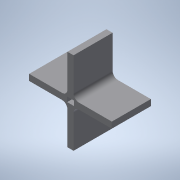
# Autodesk Inventor part: windmillv3
Saved by Autodesk Inventor 2022 (Build 260153000, 153)
## iProperties
Created: 2021-11-28
Part Number: windmillv3
Material: Generic
Document SubType Name: Modeling
Designer: haibo
Density: 1 g/cm^3
Appearance: Default
Author: haibo
Autodesk Inventor part; units mm, degrees
ref_plane "YZ Plane" through (0, 0, 0) normal (1, 0, 0) x (0, 1, 0)
ref_plane "XZ Plane" through (0, 0, 0) normal (0, 1, 0) x (-1, 0, 0)
ref_plane "XY Plane" through (0, 0, 0) normal (0, 0, 1) x (1, 0, 0)
sketch "Sketch1" plane through (0, 0, 0) normal (0, 0, 1) x (1, 0, 0)
  circle A0 centre (0, 0) radius 7.499998
  dimension "d0" = 15
  constraints: 1 centre point, 1 coincident
  measures "d0" diameter of A0
extrude "Extrusion1" add sketch "Sketch1" along normal blind 9.99998 and the other way blind 28.10002
sketch "Sketch2" plane through (0, 0, 9.99998) normal (0, 0, 1) x (1, 0, 0)
  line L0 (-2.778125, -1.984375) -> (2.778125, -1.984375)
  line L1 (2.778125, -1.984375) -> (2.778125, 1.984375)
  line L2 (2.778125, 1.984375) -> (-2.778125, 1.984375)
  line L3 (-2.778125, 1.984375) -> (-2.778125, -1.984375)
  line L4 (-2.778125, -1.984375) -> (2.778125, 1.984375) construction
  line L5 (2.778125, -1.984375) -> (-2.778125, 1.984375) construction
  point P0 (0, 0)
  dimension "d3" = 5.55625
  dimension "d4" = 3.96875
  constraints: 12 end point, 2 midpoint, 2 parallel, 1 horizontal, 1 perpendicular
  measures "d3" distance of L2.end L1.end
  measures "d4" distance of L1.end L0.end
extrude "Extrusion2" cut sketch "Sketch2" against normal blind 7.9375
ref_plane "Work Plane1" through (0, 0, 0) normal (0, 1, 0) x (0, 0, 1)
ref_plane "Work Plane2" through (0, 0, 0) normal (-1, 0, 0) x (0, 0, 1)
sketch "Sketch3" plane through (0, 0, 0) normal (0, 1, 0) x (0, 0, 1)
  point P0 (0, 0)
ref_plane "Work Plane3" through (0, 7.499998, 0) normal (0, 1, 0) x (-1, 0, 0)
ref_plane "Work Plane4" through (0, -7.499998, 0) normal (0, 1, 0) x (-1, 0, 0)
ref_plane "Work Plane5" through (-7.499998, 0, 0) normal (-1, 0, 0) x (0, -1, 0)
ref_plane "Work Plane6" through (7.499998, 0, 0) normal (-1, 0, 0) x (0, -1, 0)
sketch "Sketch4" plane through (0, 7.499998, 0) normal (0, 1, 0) x (-1, 0, 0)
  point P0 (0, 0)
sketch "Sketch5" plane through (0, 7.499998, 0) normal (0, 1, 0) x (-1, 0, 0)
  line L0 (7.499998, 9.99998) -> (-7.499998, 9.99998)
  line L1 (-2.534779, 9.99998) -> (2.534779, 9.99998)
  line L2 (2.534779, 9.99998) -> (2.534779, -28.099834)
  line L3 (2.534779, -28.099834) -> (-2.534779, -28.099834)
  line L4 (-2.534779, -28.099834) -> (-2.534779, 9.99998)
  point P0 (0, 0)
  constraints: 8 end point, 2 parallel, 2 point on line, 1 perpendicular
sketch "Sketch6" plane through (7.499998, 0, 0) normal (-1, 0, 0) x (0, -1, 0)
  line L0 (-2.534779, 9.99998) -> (2.534779, 9.99998)
  line L1 (2.534779, 9.99998) -> (2.534779, -28.099834)
  line L2 (2.534779, -28.099834) -> (-2.534779, -28.099834)
  line L3 (-2.534779, -28.099834) -> (-2.534779, 9.99998)
  point P0 (0, 0)
  constraints: 8 end point, 2 parallel, 1 perpendicular
sketch "Sketch7" plane through (0, -7.499998, 0) normal (0, 1, 0) x (-1, 0, 0)
  point P0 (0, 0)
sketch "Sketch8" plane through (0, -7.499998, 0) normal (0, 1, 0) x (-1, 0, 0)
  line L0 (-2.534779, 9.99998) -> (2.534779, 9.99998)
  line L1 (2.534779, 9.99998) -> (2.534779, -28.099834)
  line L2 (2.534779, -28.099834) -> (-2.534779, -28.099834)
  line L3 (-2.534779, -28.099834) -> (-2.534779, 9.99998)
  point P0 (0, 0)
  constraints: 8 end point, 2 parallel, 1 perpendicular
sketch "Sketch9" plane through (0, -7.499998, 0) normal (0, 1, 0) x (-1, 0, 0)
  point P0 (0, 0)
sketch "Sketch10" plane through (-7.499998, 0, 0) normal (-1, 0, 0) x (0, -1, 0)
  line L0 (7.499998, 9.99998) -> (-7.499998, 9.99998)
  line L1 (-2.542169, 9.99998) -> (2.537831, 9.99998)
  line L2 (2.537831, 9.99998) -> (2.537831, -28.10002)
  line L3 (2.537831, -28.10002) -> (-2.542169, -28.10002)
  line L4 (-2.542169, -28.10002) -> (-2.542169, 9.99998)
  point P0 (0, 0)
  dimension "d9" = 5.08
  dimension "d10" = 38.1
  constraints: 8 end point, 2 parallel, 2 point on line, 1 perpendicular
  measures "d9" distance of L1.start L1.end
  measures "d10" distance of L1.end L2.end
extrude "Extrusion3" add sketch "Sketch5" along normal blind 26.67 and the other way blind 1.27
extrude "Extrusion4" add sketch "Sketch6" along normal blind 1.27 and the other way blind 26.67
extrude "Extrusion5" add sketch "Sketch10" along normal blind 26.67 and the other way blind 1.27
extrude "Extrusion6" add sketch "Sketch8" along normal blind 1.27 and the other way blind 26.67
sketch "Sketch11" plane through (0, 0, 9.99998) normal (0, 0, 1) x (1, 0, 0)
  line L0 (2.534779, 7.058673) -> (2.534779, 6.979779)
  line L1 (34.169998, 2.534779) -> (7.058673, 2.534779)
  line L2 (6.979779, 2.534779) -> (7.058673, 2.534779)
  arc A0 (2.534779, 6.979779) -> (6.979779, 2.534779) centre (6.979779, 6.979779) ccw
  arc A1 (7.058673, 2.534779) -> (2.534779, 7.058673) centre (0, 0) ccw
  arc A2 (7.058673, 2.534779) -> (2.534779, 7.058673) centre (0, 0) ccw
  arc A3 (-2.534779, 7.058673) -> (-7.058673, 2.534779) centre (0, 0) ccw
  arc A4 (-6.979779, 2.534779) -> (-2.534779, 6.979779) centre (-6.979779, 6.979779) ccw
  line L3 (-7.058673, 2.534779) -> (-6.979779, 2.534779)
  line L4 (-2.534779, 6.979779) -> (-2.534779, 7.058673)
  arc A5 (-7.058673, -2.534779) -> (-2.534779, -7.058673) centre (0, 0) ccw
  arc A6 (-2.534779, -6.979779) -> (-6.979779, -2.534779) centre (-6.979779, -6.979779) ccw
  line L5 (-2.534779, -7.058673) -> (-2.534779, -6.979779)
  line L6 (-6.979779, -2.534779) -> (-7.058673, -2.534779)
  arc A7 (2.534779, -7.058673) -> (7.058673, -2.534779) centre (0, 0) ccw
  arc A8 (6.979779, -2.534779) -> (2.534779, -6.979779) centre (6.979779, -6.979779) ccw
  line L7 (7.058673, -2.534779) -> (6.979779, -2.534779)
  line L8 (2.534779, -6.979779) -> (2.534779, -7.058673)
  dimension "d29" = 4.445
  dimension "d32" = 360
  constraints: 16 end point, 16 point on circle, 8 centre point, 2 perpendicular, 2 tangent, 1 concentric, 41 other
  measures "d29" radius of A0
extrude "Extrusion7" cut sketch "Sketch11" against normal blind 38.1
sketch "Sketch12" plane through (0, 0, -28.10002) normal (0, 0, -1) x (-1, 0, 0)
  line L0 (2.534779, 7.058673) -> (2.534779, 34.169998)
  line L1 (-2.534779, 34.169998) -> (2.534779, 34.169998)
  line L2 (-2.534779, 7.058673) -> (-2.534779, 34.169998)
  arc A0 (-6.979779, 2.534779) -> (-2.534779, 6.979779) centre (-6.979779, 6.979779) ccw
  line L3 (-34.169998, 2.534779) -> (-7.058673, 2.534779)
  line L4 (-34.169998, -2.534779) -> (-34.169998, 2.534779)
  line L5 (-34.169998, -2.534779) -> (-7.058673, -2.534779)
  arc A1 (-2.534779, -6.979779) -> (-6.979779, -2.534779) centre (-6.979779, -6.979779) ccw
  line L6 (-2.534779, -34.169998) -> (-2.534779, -7.058673)
  line L7 (2.534779, -34.169998) -> (-2.534779, -34.169998)
  line L8 (2.534779, -34.169998) -> (2.534779, -7.058673)
  arc A2 (6.979779, -2.534779) -> (2.534779, -6.979779) centre (6.979779, -6.979779) ccw
  line L9 (7.057576, -2.537831) -> (34.169998, -2.537831)
  line L10 (34.169998, 2.542169) -> (34.169998, -2.537831)
  line L11 (7.056015, 2.542169) -> (34.169998, 2.542169)
  arc A3 (2.534779, 6.979779) -> (6.979779, 2.534779) centre (6.979779, 6.979779) ccw
  point P0 (0, 0)
extrude "Extrusion8" cut sketch "Sketch12" against normal blind 5.842 fills toward (2.484779, 20.614335) open curves L0 L1 L2
sketch "Sketch13" plane through (34.169998, 2.534779, -28.099834) normal (0, 0, -1) x (-1, 0, 0)
  line L0 (0, 0) -> (27.111325, 0)
  arc A0 (27.111325, 0) -> (27.111325, -5.069558) centre (34.169998, -2.534779) ccw
  line L1 (0, 0) -> (27.111325, 0)
  line L2 (0, -5.069558) -> (0, 0)
  line L3 (0, -5.069558) -> (27.111325, -5.069558)
  line L4 (31.635219, -9.514558) -> (31.635219, 4.445)
  arc A1 (27.190219, 0) -> (31.635219, 4.445) centre (27.190219, 4.445) ccw
  line L5 (27.190219, 0) -> (27.111325, 0)
  arc A2 (27.111325, 0) -> (27.111325, -5.069558) centre (34.169998, -2.534779) ccw
  line L6 (27.111325, -5.069558) -> (27.190219, -5.069558)
  arc A3 (31.635219, -9.514558) -> (27.190219, -5.069558) centre (27.190219, -9.514558) ccw
  line L7 (36.704777, 4.445) -> (36.704777, -9.514558)
  arc A4 (41.149777, -5.069558) -> (36.704777, -9.514558) centre (41.149777, -9.514558) ccw
  line L8 (41.149777, -5.069558) -> (41.22867, -5.069558)
  arc A5 (41.227574, -5.07261) -> (41.22867, -5.069558) centre (34.169998, -2.534779) ccw
  line L9 (41.227574, -5.07261) -> (68.339995, -5.07261)
  line L10 (68.339995, 0.00739) -> (68.339995, -5.07261)
  line L11 (41.226012, 0.00739) -> (68.339995, 0.00739)
  arc A6 (41.22867, 0) -> (41.226012, 0.00739) centre (34.169998, -2.534779) ccw
  line L12 (41.22867, 0) -> (41.149777, 0)
  arc A7 (36.704777, 4.445) -> (41.149777, 0) centre (41.149777, 4.445) ccw
extrude "Extrusion9" cut sketch "Sketch13" along normal blind 3.048 and the other way blind 5.842
body "Solid1"
